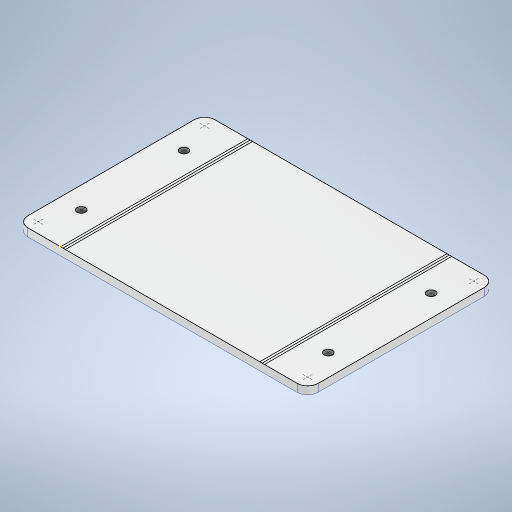
# Autodesk Inventor part: CAM_ㄷ_frame_3
Saved by Autodesk Inventor 2023 (Build 270158000, 158)
## iProperties
Created: 2022-10-29
Part Number: CAM_ㄷ_frame_3
Material: Aluminum 6061
Document SubType Name: Sheet Metal
Designer: chanh
Density: 2.7 g/cm^3
Sheet Metal Rule: Default_mm
Appearance: Aluminum - Flat
Author: chanh
Autodesk Inventor part; units mm, degrees
ref_plane "YZ Plane" through (0, 0, 0) normal (1, 0, 0) x (0, 1, 0)
ref_plane "XZ Plane" through (0, 0, 0) normal (0, 1, 0) x (-1, 0, 0)
ref_plane "XY Plane" through (0, 0, 0) normal (0, 0, 1) x (1, 0, 0)
sketch "Sketch1" plane through (0, 0, 0) normal (0, 1, 0) x (-1, 0, 0)
  line L0 (-0.4496, -35.5) -> (-0.4496, 0)
  line L1 (-38.2289, 0) -> (-38.2289, -35.5)
  circle A0 centre (-42.7736, -8) radius 0.7835
  circle A1 centre (-42.7736, -27.5) radius 0.7835
  circle A2 centre (4.095, -27.5) radius 0.7835
  circle A3 centre (4.095, -8) radius 0.7835
  arc A4 (-44.8686, 0) -> (-46.8686, -2) centre (-44.8686, -2) ccw
  line L2 (-46.8686, -33.5) -> (-46.8686, -2)
  arc A5 (-46.8686, -33.5) -> (-44.8686, -35.5) centre (-44.8686, -33.5) ccw
  arc A6 (8.19, -2) -> (6.19, 0) centre (6.19, -2) ccw
  line L3 (-44.8686, 0) -> (6.19, 0)
  arc A7 (6.19, -35.5) -> (8.19, -33.5) centre (6.19, -33.5) ccw
  line L4 (6.19, -35.5) -> (-44.8686, -35.5)
  line L5 (8.19, -2) -> (8.19, -33.5)
  line L6 (-38.6786, -35.5) -> (-38.6786, 0)
  line L7 (-37.7793, 0) -> (-37.7793, -35.5)
  line L8 (-0.8993, -35.5) -> (-0.8993, 0)
  line L9 (0, 0) -> (0, -35.5)
  point P0 (0, 0)
  constraints: 20 end point, 12 point on line, 8 centre point, 8 point on circle, 8 tangent, 8 vertical, 7 parallel, 6 equal radius, 2 horizontal, 2 perpendicular, 37 other
extrude "Plate1" add sketch "Sketch1" against normal blind 1.5
equation "\"d0\" = Thickness"
equation "\"BendReliefWidth\" = Thickness"
equation "\"BendReliefDepth\" = 0.5 * Thickness"
equation "\"CornerReliefSize\" = 4 * Thickness"
equation "\"MinimumRemnant\" = 2 * Thickness"
equation "\"TransitionRadius\" = BendRadius"
equation "\"JacobiRadiusSize\" = BendRadius"
equation "\"GapSize\" = Thickness"
equation "\"Thickness\" = 1.5"
equation "\"BendRadius\" = 0.31"
body "Solid1"
